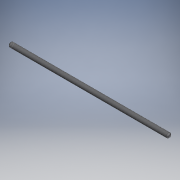
# Autodesk Inventor part: VARILLA ROSCADA
Saved by Autodesk Inventor 2018.3 (Build 223284000, 284)
## iProperties
Created: 2021-05-05
Part Number: VARILLA ROSCADA
Material: Genérico
Document SubType Name: Modeling
Designer: laguerre
Density: 8.47 g/cm^3
Appearance: Valor por defecto
Author: laguerre
Autodesk Inventor part; units mm, degrees
ref_plane "YZ Plane" through (0, 0, 0) normal (1, 0, 0) x (0, 1, 0)
ref_plane "XZ Plane" through (0, 0, 0) normal (0, 1, 0) x (-1, 0, 0)
ref_plane "XY Plane" through (0, 0, 0) normal (0, 0, 1) x (1, 0, 0)
sketch "Boceto40" plane through (0, 0, 0) normal (1, 0, 0) x (0, 1, 0)
  line L0 (0, 0) -> (0, 36.8466)
  line L1 (0, 140) -> (2, 140)
  line L2 (2, 140) -> (2, 0)
  line L3 (2, 0) -> (0, 0)
  line L4 (0, 140) -> (0, 0)
  dimension "d373" = 4
  dimension "d374" = 140
  constraints: 10 end point, 2 perpendicular, 1 collinear, 1 horizontal, 1 point on line, 1 vertical
  measures "d373" diameter of L2 L0
  measures "d374" distance of L1.end L2.end
revolve "Revolución14" add sketch "Boceto40" angle 360 about axis through (0, 0, 0) along (0, 0, 1)
thread "Rosca6" size "M4x0.7" class "6g" standard "ANSI Metric M Profile" full length
chamfer "Chaflán5" distance 1 angle 45 2 edges at (0, -2, 0) (0, -2, 140)
